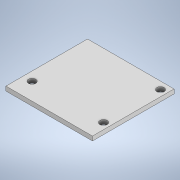
# Autodesk Inventor part: PCB_model_2
Saved by Autodesk Inventor 2020 (Build 240168000, 168)
## iProperties
Created: 2020-02-18
Part Number: PCB_model_2
Material: Generic
Document SubType Name: Modeling
Designer: nicva
Density: 1 g/cm^3
Appearance: Default
Author: nicva
Autodesk Inventor part; units mm, degrees
ref_plane "YZ Plane" through (0, 0, 0) normal (1, 0, 0) x (0, 1, 0)
ref_plane "XZ Plane" through (0, 0, 0) normal (0, 1, 0) x (-1, 0, 0)
ref_plane "XY Plane" through (0, 0, 0) normal (0, 0, 1) x (1, 0, 0)
sketch "Sketch1" plane through (0, 0, 0) normal (0, 1, 0) x (-1, 0, 0)
  line L0 (0, 0) -> (0, -33.655)
  line L1 (0, -33.655) -> (35.687, -33.655)
  line L2 (35.687, -33.655) -> (35.687, 0)
  line L3 (35.687, 0) -> (0, 0)
  line L4 (0, -33.655) -> (2.54, -33.655)
  line L5 (2.54, -33.655) -> (2.54, -30.607)
  circle A0 centre (2.54, -30.607) radius 1.5113
  line L6 (2.54, -30.607) -> (2.54, -7.112)
  circle A1 centre (2.54, -7.112) radius 1.5113
  line L7 (2.54, -7.112) -> (32.004, -7.112)
  circle A2 centre (32.004, -7.112) radius 1.5113
  dimension "d15" = 33.655
  dimension "d16" = 35.687
  dimension "d17" = 2.54
  dimension "d18" = 3.048
  dimension "d19" = 3.0226
  dimension "d20" = 23.495
  dimension "d21" = 29.464
  dimension "d22" = 3.0226
  constraints: 16 end point, 4 perpendicular, 3 centre point, 3 coincident, 2 vertical, 1 horizontal, 1 point on line
  measures "d15" distance of L0.start L0.end
  measures "d16" distance of L0.end L1.end
  measures "d17" distance of L0.end L4.end
  measures "d18" distance of L4.end L5.end
  measures "d19" diameter of A0
  measures "d20" distance of L6.start L6.end
  measures "d21" distance of L7.start L7.end
  measures "d22" diameter of A2
extrude "Extrusion2" add sketch "Sketch1" along normal blind 1.778
body "Solid2"
